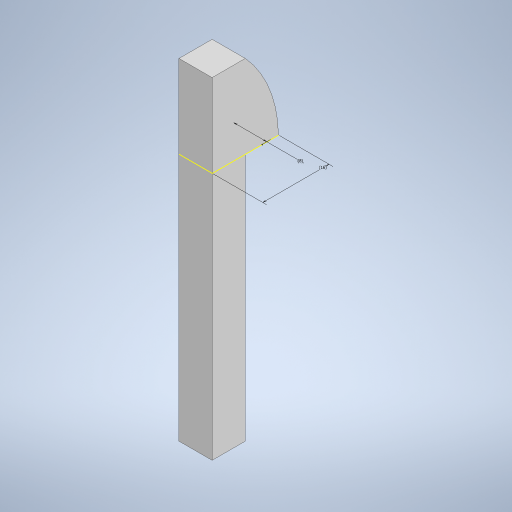
# Autodesk Inventor part: 탄두조절자
Saved by Autodesk Inventor 2023 (Build 270158000, 158)
## iProperties
Created: 2023-10-30
Part Number: 탄두조절자
Material: 일반
Document SubType Name: Modeling
Designer: rlatk
Density: 1 g/cm^3
Appearance: 기본값
Author: rlatk
Autodesk Inventor part; units mm, degrees
ref_plane "YZ Plane" through (0, 0, 0) normal (1, 0, 0) x (0, 1, 0)
ref_plane "XZ Plane" through (0, 0, 0) normal (0, 1, 0) x (-1, 0, 0)
ref_plane "XY Plane" through (0, 0, 0) normal (0, 0, 1) x (1, 0, 0)
sketch "스케치1" plane through (0, 0, 0) normal (0, 1, 0) x (-1, 0, 0)
  line L0 (0, 0) -> (-18, 0)
  line L1 (-18, 0) -> (-18, 16)
  line L2 (-18, 16) -> (0, 16)
  line L3 (0, 16) -> (0, 0)
  dimension "d0" = 18
  dimension "d1" = 16
  constraints: 8 end point, 2 parallel, 1 horizontal, 1 perpendicular
  measures "d0" distance of L1.end L2.end
  measures "d1" distance of L0.end L1.end
extrude "돌출1" add sketch "스케치1" along normal blind 40
sketch "스케치2" plane through (0, 40, 0) normal (0, 1, 0) x (1, 0, 0)
  line L0 (0, -16) -> (18, -16) projected
  line L1 (18, -16) -> (0, -16)
  line L2 (0, -16) -> (0, 8)
  line L3 (0, 8) -> (18, 8)
  line L4 (18, 8) -> (18, -16)
  point P0 (0, 0)
  dimension "d4" = 24
  constraints: 8 end point, 2 parallel, 1 horizontal, 1 perpendicular
  measures "d4" distance of L1.end L2.end
extrude "돌출2" add sketch "스케치2" along normal blind 20
sketch "스케치3" plane through (0, 0, 0) normal (-1, 0, 0) x (0, 0, 1)
  line L0 (-8, 40) -> (-8, 60) projected
  arc A0 (0, 60) -> (-8, 40) centre (22.4205, 39.4318) ccw
  line L1 (0, 40) -> (-8, 40) projected
  line L2 (-8, 40) -> (-8, 60)
  line L3 (16, 60) -> (-8, 60) projected
  line L4 (-8, 60) -> (0, 60)
  point P0 (0, 0)
  constraints: 4 end point, 3 point on circle, 1 centre point, 1 collinear, 1 perpendicular
extrude "돌출3" cut sketch "스케치3" against normal blind 20
sketch "스케치4" plane through (0, 60, 0) normal (0, 1, 0) x (1, 0, 0)
  line L0 (0, -16) -> (18, -16) projected
  line L1 (18, -16) -> (18, 0) projected
  line L2 (0, -16) -> (18, -16)
  line L3 (18, -16) -> (18, -8)
  line L4 (18, -8) -> (0, -8)
  line L5 (0, -8) -> (0, -16)
  point P0 (0, 0)
  constraints: 8 end point, 2 parallel, 1 horizontal, 1 midpoint, 1 perpendicular
extrude "돌출4" cut sketch "스케치4" against normal blind 60
sketch "스케치5" plane through (0, 60, 8) normal (0, 0, 1) x (1, 0, 0)
  line L0 (0, 0) -> (18, 0) projected
  line L1 (0, -60) -> (0, 0) projected
  line L2 (18, -60) -> (0, -60) projected
  line L3 (18, 0) -> (18, -60) projected
  line L4 (18, -60) -> (8, -60)
  line L5 (8, -60) -> (8, 0)
  line L6 (8, 0) -> (18, 0)
  line L7 (18, 0) -> (18, -60)
  point P0 (0, -60)
  dimension "d11" = 10
  constraints: 8 end point, 2 parallel, 1 horizontal, 1 perpendicular, 1 point on line
  measures "d11" distance of L5.end L6.end
extrude "돌출5" cut sketch "스케치5" against normal blind 60 contours L0 L3 L2 L5
sketch "스케치6" plane through (0, 0, 0) normal (0, -1, 0) x (1, 0, 0)
  line L0 (0, 0) -> (0, 8) projected
  line L1 (0, 8) -> (8, 8) projected
  line L2 (0, 0) -> (8, 0)
  line L3 (8, 0) -> (8, 8)
  line L4 (8, 8) -> (0, 8)
  line L5 (0, 8) -> (0, 0)
  constraints: 8 end point, 2 parallel, 1 horizontal, 1 perpendicular
extrude "돌출6" add sketch "스케치6" along normal blind 20
sketch "스케치7" plane through (0, 40, 0) normal (0, -1, 0) x (1, 0, 0)
  line L0 (8, -8) -> (8, 0) projected
  line L1 (8, 0) -> (0, 0) projected
  line L2 (0, -8) -> (0, 0) projected
  line L3 (8, -8) -> (0, -8) projected
  line L4 (8, 8) -> (0, 8) projected
  line L5 (0, 8) -> (0, 0) projected
  line L6 (0, 0) -> (8, 0) projected
  line L7 (8, 0) -> (8, 8) projected
  point P0 (8, -4)
  dimension "d16" = 8
  dimension "d17" = 16
  constraints: 1 midpoint
  measures "d16" distance from line of point (8, -4) L2
  measures "d17" distance between parallel lines of L4 L3
